Autodesk Inventor part; units mm, degrees
(part 2 of 2)
  arc A140 (-25.4446, 74.7133) -> (-26.798, 74.2336) centre (-25.1834, 71.8276) ccw
  arc A141 (-26.798, 74.2336) -> (-27.2062, 73.5932) centre (-26.3001, 73.4659) ccw
  arc A142 (-21.4794, 73.1947) -> (-22.0085, 74.2336) centre (-22.7699, 73.1916) ccw
  circle A143 centre (-25.9605, 73.338) radius 0.5161
  line L110 (-27.2062, 73.5932) -> (-27.2062, 72.1245)
  line L111 (-27.2062, 72.1245) -> (-24.3395, 72.1245)
  line L112 (-24.3395, 71.7056) -> (-28.3839, 71.7056)
  line L113 (-24.3395, 72.1245) -> (-24.3395, 71.7056)
  line L114 (-21.4733, 70.5884) -> (-21.4794, 73.1947)
  arc A144 (-23.3243, 25.8454) -> (-25.4322, 25.8454) centre (-24.3782, 17.6506) ccw
  arc A145 (-25.4322, 25.8454) -> (-26.7856, 25.3656) centre (-25.171, 22.9597) ccw
  arc A146 (-21.9961, 25.3656) -> (-23.3243, 25.8454) centre (-23.7019, 22.7218) ccw
  arc A147 (-21.4671, 24.3267) -> (-21.9961, 25.3656) centre (-22.7575, 24.3237) ccw
  arc A148 (-26.7856, 25.3656) -> (-27.1938, 24.7252) centre (-26.2877, 24.5979) ccw
  circle A149 centre (-25.9607, 24.5305) radius 0.545
  line L115 (-27.1938, 24.7252) -> (-27.1938, 23.2566)
  line L116 (-27.1938, 23.2566) -> (-24.3272, 23.2566)
  line L117 (-24.3272, 23.2566) -> (-24.3272, 22.8376)
  line L118 (-21.461, 21.7204) -> (-21.4671, 24.3267)
  line L119 (-26.0801, 20.1743) -> (-23.0926, 20.1813)
  arc A150 (-22.5618, 19.8544) -> (-21.3196, 20.5365) centre (-22.5875, 21.3734) ccw
  arc A151 (-23.0926, 20.1813) -> (-21.461, 21.7204) centre (-22.9431, 21.6573) ccw
  line L120 (-22.5618, 19.8544) -> (-25.5493, 19.8474)
  line L121 (-21.0597, 22.9429) -> (-21.0597, 21.4689)
  arc A152 (-21.3196, 20.5365) -> (-21.0597, 21.4689) centre (-22.9439, 21.4916) ccw
  line L122 (-19.9288, 22.9429) -> (-21.0597, 22.9429)
  arc A153 (-18.7198, 21.9341) -> (-19.9288, 22.9429) centre (-20.2582, 21.3193) ccw
  arc A154 (-18.5273, 18.7011) -> (-18.7198, 21.9341) centre (-23.4893, 20.0279) ccw
  arc A155 (-20.2704, 17.1911) -> (-18.5273, 18.7011) centre (-20.3549, 19.0497) ccw
  arc A156 (-25.5493, 19.8474) -> (-27.181, 18.3083) centre (-25.6988, 18.3715) ccw
  arc A157 (-26.0801, 20.1743) -> (-27.3224, 19.4922) centre (-26.0545, 18.6554) ccw
  line L123 (-24.3272, 22.8376) -> (-28.3715, 22.8376)
  arc A158 (-27.3224, 19.4922) -> (-27.5822, 18.5598) centre (-25.698, 18.5371) ccw
  line L124 (-27.5822, 17.0858) -> (-27.5822, 18.5598)
  arc A159 (-28.3715, 22.8376) -> (-30.1146, 21.3277) centre (-28.287, 20.979) ccw
  line L125 (-28.7131, 17.0858) -> (-27.5822, 17.0858)
  arc A160 (-30.1146, 21.3277) -> (-29.9221, 18.0946) centre (-25.1526, 20.0009) ccw
  arc A161 (-29.9221, 18.0946) -> (-28.7131, 17.0858) centre (-28.3837, 18.7095) ccw
  arc A162 (-25.3176, 14.1834) -> (-23.2097, 14.1834) centre (-24.2637, 22.3782) ccw
  arc A163 (-26.6458, 14.6631) -> (-25.3176, 14.1834) centre (-24.94, 17.307) ccw
  arc A164 (-23.2097, 14.1834) -> (-21.8563, 14.6631) centre (-23.4709, 17.0691) ccw
  arc A165 (-21.8563, 14.6631) -> (-21.4481, 15.3035) centre (-22.3542, 15.4308) ccw
  arc A166 (-27.1749, 15.702) -> (-26.6458, 14.6631) centre (-25.8844, 15.705) ccw
  circle A167 centre (-22.6938, 15.5587) radius 0.5161
  line L126 (-21.4481, 15.3035) -> (-21.4481, 16.7721)
  line L127 (-21.4481, 16.7721) -> (-24.3148, 16.7721)
  line L128 (-24.3148, 17.1911) -> (-20.2704, 17.1911)
  line L129 (-24.3148, 16.7721) -> (-24.3148, 17.1911)
  line L130 (-27.181, 18.3083) -> (-27.1749, 15.702)
  arc A168 (-32.7529, 38.6055) -> (-30.645, 38.6055) centre (-31.6989, 46.8003) ccw
  arc A169 (-30.645, 38.6055) -> (-29.2915, 39.0853) centre (-30.9061, 41.4912) ccw
  arc A170 (-34.081, 39.0853) -> (-32.7529, 38.6055) centre (-32.3753, 41.7291) ccw
  arc A171 (-34.6101, 40.1242) -> (-34.081, 39.0853) centre (-33.3196, 40.1272) ccw
  arc A172 (-29.2915, 39.0853) -> (-28.8833, 39.7256) centre (-29.7895, 39.853) ccw
  circle A173 centre (-30.1164, 39.9204) radius 0.545
  line L131 (-28.8833, 39.7256) -> (-28.8833, 41.1943)
  line L132 (-28.8833, 41.1943) -> (-31.75, 41.1943)
  line L133 (-31.75, 41.1943) -> (-31.75, 41.6132)
  line L134 (-34.6162, 42.7305) -> (-34.6101, 40.1242)
  line L135 (-29.9971, 44.2766) -> (-32.9846, 44.2696)
  arc A174 (-33.5153, 44.5964) -> (-34.7576, 43.9143) centre (-33.4897, 43.0775) ccw
  arc A175 (-32.9846, 44.2696) -> (-34.6162, 42.7305) centre (-33.134, 42.7936) ccw
  line L136 (-33.5153, 44.5964) -> (-30.5278, 44.6034)
  line L137 (-35.0174, 41.508) -> (-35.0174, 42.982)
  arc A176 (-34.7576, 43.9143) -> (-35.0174, 42.982) centre (-33.1333, 42.9593) ccw
  line L138 (-36.1484, 41.508) -> (-35.0174, 41.508)
  arc A177 (-37.3573, 42.5167) -> (-36.1484, 41.508) centre (-35.819, 43.1316) ccw
  arc A178 (-37.5499, 45.7498) -> (-37.3573, 42.5167) centre (-32.5879, 44.423) ccw
  arc A179 (-35.8068, 47.2598) -> (-37.5499, 45.7498) centre (-35.7223, 45.4011) ccw
  arc A180 (-30.5278, 44.6034) -> (-28.8962, 46.1426) centre (-30.3784, 46.0794) ccw
  arc A181 (-29.9971, 44.2766) -> (-28.7548, 44.9587) centre (-30.0227, 45.7955) ccw
  line L139 (-31.75, 41.6132) -> (-27.7056, 41.6132)
  arc A182 (-28.7548, 44.9587) -> (-28.495, 45.891) centre (-30.3791, 45.9137) ccw
  line L140 (-28.495, 47.365) -> (-28.495, 45.891)
  arc A183 (-27.7056, 41.6132) -> (-25.9625, 43.1232) centre (-27.7901, 43.4719) ccw
  line L141 (-27.364, 47.365) -> (-28.495, 47.365)
  arc A184 (-25.9625, 43.1232) -> (-26.155, 46.3563) centre (-30.9245, 44.45) ccw
  arc A185 (-26.155, 46.3563) -> (-27.364, 47.365) centre (-27.6934, 45.7414) ccw
  arc A186 (-30.7595, 50.2675) -> (-32.8674, 50.2675) centre (-31.8135, 42.0727) ccw
  arc A187 (-29.4314, 49.7878) -> (-30.7595, 50.2675) centre (-31.1371, 47.1439) ccw
  arc A188 (-32.8674, 50.2675) -> (-34.2209, 49.7878) centre (-32.6063, 47.3818) ccw
  arc A189 (-34.2209, 49.7878) -> (-34.6291, 49.1474) centre (-33.7229, 49.02) ccw
  arc A190 (-28.9023, 48.7488) -> (-29.4314, 49.7878) centre (-30.1928, 48.7458) ccw
  circle A191 centre (-33.3833, 48.8922) radius 0.5161
  line L142 (-34.6291, 49.1474) -> (-34.6291, 47.6787)
  line L143 (-34.6291, 47.6787) -> (-31.7624, 47.6787)
  line L144 (-31.7624, 47.2598) -> (-35.8068, 47.2598)
  line L145 (-31.7624, 47.6787) -> (-31.7624, 47.2598)
  line L146 (-28.8962, 46.1426) -> (-28.9023, 48.7488)
  spline S0 degree 2 poles (-50.6604, 78.8056) (-50.6604, 78.0729) (-51.1297, 76.8214) (-51.5579, 76.3603) knots 0 0 0 1 2 2 2
  spline S1 degree 2 poles (-51.5579, 76.3603) (-51.986, 75.8992) (-53.2622, 75.3641) (-54.0526, 75.3641) knots 0 0 0 1 2 2 2
  spline S2 degree 2 poles (-54.0526, 75.3641) (-54.7771, 75.3641) (-56.1933, 75.6852) (-56.712, 75.9404) knots 0 0 0 1 2 2 2
  line L147 (-56.712, 75.9404) -> (-56.712, 77.3813)
  line L148 (-56.712, 77.3813) -> (-56.6132, 77.3813)
  spline S3 degree 2 poles (-56.6132, 77.3813) (-56.4567, 77.266) (-55.8722, 76.9696) (-55.5181, 76.8379) knots 0 0 0 1 2 2 2
  spline S4 degree 2 poles (-55.5181, 76.8379) (-55.1147, 76.6979) (-54.4478, 76.5415) (-54.0279, 76.5415) knots 0 0 0 1 2 2 2
  spline S5 degree 2 poles (-54.0279, 76.5415) (-53.6162, 76.5415) (-52.8423, 76.8379) (-52.5623, 77.159) knots 0 0 0 1 2 2 2
  spline S6 degree 2 poles (-52.5623, 77.159) (-52.3071, 77.4636) (-52.0436, 78.2705) (-52.0436, 78.8139) knots 0 0 0 1 2 2 2
  spline S7 degree 2 poles (-52.0436, 78.8139) (-52.0436, 79.3573) (-52.34, 80.0489) (-52.62, 80.2794) knots 0 0 0 1 2 2 2
  spline S8 degree 2 poles (-52.62, 80.2794) (-52.9081, 80.5346) (-53.7644, 80.7487) (-54.2831, 80.7487) knots 0 0 0 1 2 2 2
  spline S9 degree 2 poles (-54.2831, 80.7487) (-54.843, 80.7487) (-55.9545, 80.5758) (-56.2921, 80.5017) knots 0 0 0 1 2 2 2
  line L149 (-56.2921, 80.5017) -> (-56.2921, 85.7381)
  line L150 (-56.2921, 85.7381) -> (-50.7181, 85.7381)
  line L151 (-50.7181, 85.7381) -> (-50.7181, 84.5443)
  line L152 (-50.7181, 84.5443) -> (-54.9829, 84.5443)
  line L153 (-54.9829, 84.5443) -> (-54.9829, 81.8355)
  spline S10 degree 2 poles (-54.9829, 81.8355) (-54.7359, 81.8685) (-54.2584, 81.8932) (-54.0608, 81.8932) knots 0 0 0 1 2 2 2
  spline S11 degree 2 poles (-54.0608, 81.8932) (-53.2786, 81.8932) (-52.2001, 81.6379) (-51.7061, 81.2592) knots 0 0 0 1 2 2 2
  spline S12 degree 2 poles (-51.7061, 81.2592) (-51.2038, 80.8804) (-50.6604, 79.7278) (-50.6604, 78.8056) knots 0 0 0 1 2 2 2
  spline S13 degree 2 poles (-12.8396, 10.4389) (-12.8396, 11.1717) (-12.3703, 12.4232) (-11.9421, 12.8843) knots 0 0 0 1 2 2 2
  spline S14 degree 2 poles (-11.9421, 12.8843) (-11.514, 13.3453) (-10.2378, 13.8805) (-9.4474, 13.8805) knots 0 0 0 1 2 2 2
  spline S15 degree 2 poles (-9.4474, 13.8805) (-8.7229, 13.8805) (-7.3067, 13.5594) (-6.788, 13.3042) knots 0 0 0 1 2 2 2
  line L154 (-6.788, 13.3042) -> (-6.788, 11.8633)
  line L155 (-6.788, 11.8633) -> (-6.8868, 11.8633)
  spline S16 degree 2 poles (-6.8868, 11.8633) (-7.0433, 11.9786) (-7.6278, 12.275) (-7.9819, 12.4067) knots 0 0 0 1 2 2 2
  spline S17 degree 2 poles (-7.9819, 12.4067) (-8.3853, 12.5467) (-9.0522, 12.7031) (-9.4721, 12.7031) knots 0 0 0 1 2 2 2
  spline S18 degree 2 poles (-9.4721, 12.7031) (-9.8838, 12.7031) (-10.6577, 12.4067) (-10.9377, 12.0856) knots 0 0 0 1 2 2 2
  spline S19 degree 2 poles (-10.9377, 12.0856) (-11.1929, 11.781) (-11.4564, 10.9741) (-11.4564, 10.4307) knots 0 0 0 1 2 2 2
  spline S20 degree 2 poles (-11.4564, 10.4307) (-11.4564, 9.8873) (-11.16, 9.1957) (-10.88, 8.9652) knots 0 0 0 1 2 2 2
  spline S21 degree 2 poles (-10.88, 8.9652) (-10.5919, 8.7099) (-9.7356, 8.4959) (-9.2169, 8.4959) knots 0 0 0 1 2 2 2
  spline S22 degree 2 poles (-9.2169, 8.4959) (-8.657, 8.4959) (-7.5455, 8.6688) (-7.2079, 8.7429) knots 0 0 0 1 2 2 2
  line L156 (-7.2079, 8.7429) -> (-7.2079, 3.5064)
  line L157 (-7.2079, 3.5064) -> (-12.7819, 3.5064)
  line L158 (-12.7819, 3.5064) -> (-12.7819, 4.7003)
  line L159 (-12.7819, 4.7003) -> (-8.5171, 4.7003)
  line L160 (-8.5171, 4.7003) -> (-8.5171, 7.4091)
  spline S23 degree 2 poles (-8.5171, 7.4091) (-8.7641, 7.3761) (-9.2416, 7.3514) (-9.4392, 7.3514) knots 0 0 0 1 2 2 2
  spline S24 degree 2 poles (-9.4392, 7.3514) (-10.2214, 7.3514) (-11.2999, 7.6067) (-11.7939, 7.9854) knots 0 0 0 1 2 2 2
  spline S25 degree 2 poles (-11.7939, 7.9854) (-12.2962, 8.3641) (-12.8396, 9.5168) (-12.8396, 10.4389) knots 0 0 0 1 2 2 2
  spline S26 degree 2 poles (-50.6604, 78.8056) (-50.6604, 78.0729) (-51.1297, 76.8214) (-51.5579, 76.3603) knots 0 0 0 1 2 2 2
  spline S27 degree 2 poles (-51.5579, 76.3603) (-51.986, 75.8992) (-53.2622, 75.3641) (-54.0526, 75.3641) knots 0 0 0 1 2 2 2
  spline S28 degree 2 poles (-54.0526, 75.3641) (-54.7771, 75.3641) (-56.1933, 75.6852) (-56.712, 75.9404) knots 0 0 0 1 2 2 2
  line L161 (-56.712, 75.9404) -> (-56.712, 77.3813)
  line L162 (-56.712, 77.3813) -> (-56.6132, 77.3813)
  spline S29 degree 2 poles (-56.6132, 77.3813) (-56.4567, 77.266) (-55.8722, 76.9696) (-55.5181, 76.8379) knots 0 0 0 1 2 2 2
  spline S30 degree 2 poles (-55.5181, 76.8379) (-55.1147, 76.6979) (-54.4478, 76.5415) (-54.0279, 76.5415) knots 0 0 0 1 2 2 2
  spline S31 degree 2 poles (-54.0279, 76.5415) (-53.6162, 76.5415) (-52.8423, 76.8379) (-52.5623, 77.159) knots 0 0 0 1 2 2 2
  spline S32 degree 2 poles (-52.5623, 77.159) (-52.3071, 77.4636) (-52.0436, 78.2705) (-52.0436, 78.8139) knots 0 0 0 1 2 2 2
  spline S33 degree 2 poles (-52.0436, 78.8139) (-52.0436, 79.3573) (-52.34, 80.0489) (-52.62, 80.2794) knots 0 0 0 1 2 2 2
  spline S34 degree 2 poles (-52.62, 80.2794) (-52.9081, 80.5346) (-53.7644, 80.7487) (-54.2831, 80.7487) knots 0 0 0 1 2 2 2
  spline S35 degree 2 poles (-54.2831, 80.7487) (-54.843, 80.7487) (-55.9545, 80.5758) (-56.2921, 80.5017) knots 0 0 0 1 2 2 2
  line L163 (-56.2921, 80.5017) -> (-56.2921, 85.7381)
  line L164 (-56.2921, 85.7381) -> (-50.7181, 85.7381)
  line L165 (-50.7181, 85.7381) -> (-50.7181, 84.5443)
  line L166 (-50.7181, 84.5443) -> (-54.9829, 84.5443)
  line L167 (-54.9829, 84.5443) -> (-54.9829, 81.8355)
  spline S36 degree 2 poles (-54.9829, 81.8355) (-54.7359, 81.8685) (-54.2584, 81.8932) (-54.0608, 81.8932) knots 0 0 0 1 2 2 2
  spline S37 degree 2 poles (-54.0608, 81.8932) (-53.2786, 81.8932) (-52.2001, 81.6379) (-51.7061, 81.2592) knots 0 0 0 1 2 2 2
  spline S38 degree 2 poles (-51.7061, 81.2592) (-51.2038, 80.8804) (-50.6604, 79.7278) (-50.6604, 78.8056) knots 0 0 0 1 2 2 2
  spline S39 degree 2 poles (-12.8396, 10.4389) (-12.8396, 11.1717) (-12.3703, 12.4232) (-11.9421, 12.8843) knots 0 0 0 1 2 2 2
  spline S40 degree 2 poles (-11.9421, 12.8843) (-11.514, 13.3453) (-10.2378, 13.8805) (-9.4474, 13.8805) knots 0 0 0 1 2 2 2
  spline S41 degree 2 poles (-9.4474, 13.8805) (-8.7229, 13.8805) (-7.3067, 13.5594) (-6.788, 13.3042) knots 0 0 0 1 2 2 2
  line L168 (-6.788, 13.3042) -> (-6.788, 11.8633)
  line L169 (-6.788, 11.8633) -> (-6.8868, 11.8633)
  spline S42 degree 2 poles (-6.8868, 11.8633) (-7.0433, 11.9786) (-7.6278, 12.275) (-7.9819, 12.4067) knots 0 0 0 1 2 2 2
  spline S43 degree 2 poles (-7.9819, 12.4067) (-8.3853, 12.5467) (-9.0522, 12.7031) (-9.4721, 12.7031) knots 0 0 0 1 2 2 2
  spline S44 degree 2 poles (-9.4721, 12.7031) (-9.8838, 12.7031) (-10.6577, 12.4067) (-10.9377, 12.0856) knots 0 0 0 1 2 2 2
  spline S45 degree 2 poles (-10.9377, 12.0856) (-11.1929, 11.781) (-11.4564, 10.9741) (-11.4564, 10.4307) knots 0 0 0 1 2 2 2
  spline S46 degree 2 poles (-11.4564, 10.4307) (-11.4564, 9.8873) (-11.16, 9.1957) (-10.88, 8.9652) knots 0 0 0 1 2 2 2
  spline S47 degree 2 poles (-10.88, 8.9652) (-10.5919, 8.7099) (-9.7356, 8.4959) (-9.2169, 8.4959) knots 0 0 0 1 2 2 2
  spline S48 degree 2 poles (-9.2169, 8.4959) (-8.657, 8.4959) (-7.5455, 8.6688) (-7.2079, 8.7429) knots 0 0 0 1 2 2 2
  line L170 (-7.2079, 8.7429) -> (-7.2079, 3.5064)
  line L171 (-7.2079, 3.5064) -> (-12.7819, 3.5064)
  line L172 (-12.7819, 3.5064) -> (-12.7819, 4.7003)
  line L173 (-12.7819, 4.7003) -> (-8.5171, 4.7003)
  line L174 (-8.5171, 4.7003) -> (-8.5171, 7.4091)
  spline S49 degree 2 poles (-8.5171, 7.4091) (-8.7641, 7.3761) (-9.2416, 7.3514) (-9.4392, 7.3514) knots 0 0 0 1 2 2 2
  spline S50 degree 2 poles (-9.4392, 7.3514) (-10.2214, 7.3514) (-11.2999, 7.6067) (-11.7939, 7.9854) knots 0 0 0 1 2 2 2
  spline S51 degree 2 poles (-11.7939, 7.9854) (-12.2962, 8.3641) (-12.8396, 9.5168) (-12.8396, 10.4389) knots 0 0 0 1 2 2 2
  point P0 (-39.1737, 68.8958)
  point P1 (-39.1737, 20.0009)
  point P2 (-53.7479, 68.8958)
  point P3 (-9.7521, 20.0042)
  point P4 (-13.4723, 102.9238)
  point P5 (-39.1737, 68.8958)
  point P6 (-39.1737, 20.0009)
  point P7 (-53.7479, 68.8958)
  point P8 (-9.7521, 20.0042)
  point P9 (-24.3263, 68.8958)
  point P10 (-24.3272, 68.8958)
  point P11 (-24.3272, 20.0009)
  point P12 (-24.3272, 68.8958)
  point P13 (-24.3272, 20.0009)
  point P14 (-31.75, 44.45)
  point P15 (-31.75, 44.45)
  point P16 (-31.75, 44.45)
  dimension "d103" = 8.4153
  dimension "d105" = 0.508
  dimension "d106" = 0.508
  constraints: 352 point on circle, 268 end point, 192 centre point, 32 perpendicular, 32 tangent, 12 vertical, 6 horizontal, 4 midpoint, 1 parallel, 1 point on line, 1 symmetric about line, 4 other
  measures "d103" distance of L12.end L14.start
  measures "d105" distance between parallel lines of L15 L7
  measures "d106" distance between parallel lines of L16 L11
extrude "Extrusion20" add sketch "Sketch17" along normal blind 0.4 contours L40 A34 A33 A32 L39 L38 L37 L36 A31 A30 A29 A28 A27 L35 A26 L34 A25 A24 L33 | L56 A58 A57 A56 L55 L54 L53 L52 A55 A54 A53 A52 A51 L51 A50 L50 A49 A48 L49 | L72 A82 A81 A80 L71 L70 L69 L68 A79 A78 A77 A76 A75 L67 A74 L66 A73 A72 L65 | L92 A113 A112 L95 L96 A116 A117 A115 L93 L89 L91 L94 A111 A110 A108 A114 A109 L90 A107 | A122 A123 L102 A127 L103 A133 A134 L108 L109 A137 A136 A135 L107 L101 L100 L99 A124 A121 A120 | A150 A152 L121 L122 A153 A154 A155 L128 L129 L127 L126 A165 A164 A162 A163 A166 L130 A156 L120 | A174 A176 L137 L138 A177 A178 A179 L144 L145 L143 L142 A189 A188 A186 A187 A190 L146 A180 L136 | S0 S1 S2 L147 L148 S3 S4 S5 S6 S7 S8 S9 L149 L150 L151 L152 L153 S10 S11 S12 | S13 S14 S15 L154 L155 S16 S17 S18 S19 S20 S21 S22 L156 L157 L158 L159 L160 S23 S24 S25 bodies 1
sketch "Sketch18" plane through (0, 0, -0.2) normal (0, 0, -1) x (-1, 0, 0)
  line L0 (0, 0) -> (-63.5, 0)
  line L1 (-63.5, 0) -> (-63.5, 88.9)
  line L2 (-63.5, 88.9) -> (0, 88.9)
  line L3 (0, 88.9) -> (0, 0)
  constraints: 8 end point, 2 parallel, 1 horizontal, 1 perpendicular
extrude "Extrusion21" add sketch "Sketch18" along normal blind 0.4 bodies 3
fillet "Fillet2" radius 3.175 8 edges at (63.5, 0, 0.2) (63.5, 88.9, 0.2) (0, 0, 0.2) (0, 88.9, 0.2) (63.5, 0, -0.3) (63.5, 88.9, -0.3) (0, 0, -0.3) (0, 88.9, -0.3)
extrude "Extrusion22" cut sketch "Sketch17" along normal blind 0.4 contours L40 A34 A33 A32 L39 L38 L37 L36 A31 A30 A29 A28 A27 L35 A26 L34 A25 A24 L33 | L44 A41 A40 L47 L48 A44 A45 A43 L45 L41 L43 L46 A39 A38 A36 A42 A37 L42 A35 | L56 A58 A57 A56 L55 L54 L53 L52 A55 A54 A53 A52 A51 L51 A50 L50 A49 A48 L49 | L60 A65 A64 L63 L64 A68 A69 A67 L61 L57 L59 L62 A63 A62 A60 A66 A61 L58 A59 | L72 A82 A81 A80 L71 L70 L69 L68 A79 A78 A77 A76 A75 L67 A74 L66 A73 A72 L65 | L76 A89 A88 L79 L80 A92 A93 A91 L77 L73 L75 L78 A87 A86 A84 A90 A85 L74 A83 | L88 A106 A105 A104 L87 L86 L85 L84 A103 A102 A101 A100 A99 L83 A98 L82 A97 A96 L81 | L92 A113 A112 L95 L96 A116 A117 A115 L93 L89 L91 L94 A111 A110 A108 A114 A109 L90 A107 | A122 A123 L102 A127 L103 A133 A134 L108 L109 A137 A136 A135 L107 L101 L100 L99 A124 A121 A120 | A126 A128 L105 L106 A129 A130 A131 L112 L113 L111 L110 A141 A140 A138 A139 A142 L114 A132 L104 | A146 A147 L118 A151 L119 A157 A158 L124 L125 A161 A160 A159 L123 L117 L116 L115 A148 A145 A144 | A150 A152 L121 L122 A153 A154 A155 L128 L129 L127 L126 A165 A164 A162 A163 A166 L130 A156 L120 | A170 A171 L134 A175 L135 A181 A182 L140 L141 A185 A184 A183 L139 L133 L132 L131 A172 A169 A168 | A174 A176 L137 L138 A177 A178 A179 L144 L145 L143 L142 A189 A188 A186 A187 A190 L146 A180 L136 | S0 S1 S2 L147 L148 S3 S4 S5 S6 S7 S8 S9 L149 L150 L151 L152 L153 S10 S11 S12 | S13 S14 S15 L154 L155 S16 S17 S18 S19 S20 S21 S22 L156 L157 L158 L159 L160 S23 S24 S25 bodies 3
extrude "Extrusion23" add sketch "Sketch17" along normal blind 0.4 contours L44 A41 A40 L47 L48 A44 A45 A43 L45 L41 L43 L46 A39 A38 A36 A42 A37 L42 A35 | L60 A65 A64 L63 L64 A68 A69 A67 L61 L57 L59 L62 A63 A62 A60 A66 A61 L58 A59 | L76 A89 A88 L79 L80 A92 A93 A91 L77 L73 L75 L78 A87 A86 A84 A90 A85 L74 A83 | L88 A106 A105 A104 L87 L86 L85 L84 A103 A102 A101 A100 A99 L83 A98 L82 A97 A96 L81 | A126 A128 L105 L106 A129 A130 A131 L112 L113 L111 L110 A141 A140 A138 A139 A142 L114 A132 L104 | A146 A147 L118 A151 L119 A157 A158 L124 L125 A161 A160 A159 L123 L117 L116 L115 A148 A145 A144 | A170 A171 L134 A175 L135 A181 A182 L140 L141 A185 A184 A183 L139 L133 L132 L131 A172 A169 A168 bodies 4
